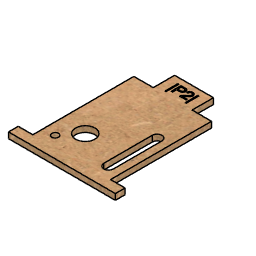
P2 (Autodesk Fusion 360 design; units mm, degrees)
Autodesk Fusion 360 part; units mm, degrees
note: some values were not read from the file. Set by a fixed rule: which sketch regions a step uses.
sketch "Esboço1" plane through (0, 0, 0) normal (0, 1, 0) x (1, 0, 0)
  line L0 (0, 0) -> (55, 0)
  line L1 (55, 0) -> (55, 5)
  line L2 (55, 5) -> (47.5, 5)
  line L3 (17.5, 68) -> (17.5, 57)
  line L4 (17.5, 57) -> (7.5, 57)
  line L5 (7.5, 57) -> (7.5, 5)
  line L6 (7.5, 5) -> (0, 5)
  line L7 (0, 5) -> (0, 0)
  circle A0 centre (13.5, 10.5) radius 1.75
  line L8 (43.5, 35.5) -> (43.5, 10.5)
  line L9 (38.5, 10.5) -> (38.5, 35.5)
  circle A1 centre (20.5, 19) radius 5
  line L10 (41, 68.4978) -> (41, 0)
  arc A2 (38.5, 10.5) -> (43.5, 10.5) centre (41, 10.5) ccw
  arc A3 (43.5, 35.5) -> (38.5, 35.5) centre (41, 35.5) ccw
  line L11 (37.5, 68) -> (37.5, 57)
  line L12 (37.5, 57) -> (47.5, 57)
  line L13 (17.5, 68) -> (37.5, 68)
  line L14 (47.5, 57) -> (47.5, 5)
  dimension "d1" = 55
  dimension "d2" = 5
  dimension "d4" = 10
  dimension "d8" = 3.5
  dimension "d10" = 6
  dimension "d18" = 10
  dimension "d38" = 5.5
  dimension "d39" = 7.5
  dimension "d41" = 11
  dimension "d42" = 52
  dimension "d45" = 20.5
  dimension "d46" = 2.5
  dimension "d47" = 5.5
  dimension "d48" = 5
  dimension "d49" = 25
  dimension "d50" = 2.5
  dimension "d51" = 8.5
  dimension "d54" = 11
  dimension "d55" = 10
  dimension "d56" = 20
  dimension "d57" = 52
  dimension "d58" = 4
  constraint coincident L0.start L7.end
  constraint horizontal L0
  constraint perpendicular L0 L1
  constraint perpendicular L1 L2
  constraint perpendicular L3 L4
  constraint perpendicular L4 L5
  constraint perpendicular L5 L6
  constraint perpendicular L0 L7
  constraint vertical L8
  constraint vertical L9
  constraint collinear L2 L6
  constraint vertical L10
  constraint coincident L0 L10.end
  constraint coincident L10 A2.centre
  constraint coincident L10 A3.centre
  constraint perpendicular L11 L13
  constraint perpendicular L2 L14
  measures "d1" distance of L0.start L0.end
  measures "d2" distance of L0.end L1.end
  measures "d4" distance of L3.end L4.end
  measures "d8" diameter of A0
  measures "d10" distance of L5 A0.centre
  measures "d18" diameter of A1
  measures "d38" distance of L6 A0.centre
  measures "d39" distance of L5.end L6.end
  measures "d41" distance of L3.start L3.end
  measures "d42" distance of L4.end L5.end
  measures "d45" distance of A1.centre L10
  measures "d46" radius of A2
  measures "d47" distance of L2 A2.centre
  measures "d48" distance of L8 L9
  measures "d49" distance of L8.end L8.start
  measures "d50" radius of A3
  measures "d51" vertical distance of A1.centre A2.centre
  measures "d54" distance of L11.start L11.end
  measures "d55" distance of L11.end L12.end
  measures "d56" distance of L3.start L11.start
  measures "d57" distance of L2 L12
  measures "d58" distance of L8 L14
extrude "Extrusão1" add sketch "Esboço1" along normal blind 3 contours L0 L3 L4 L5 L6 L7 L9 L10 A2 A3 L11 L12 L13 | L0 L1 L2 L8 L10 A2 A3 L12 L14
sketch "Esboço2" plane through (0, 3, 0) normal (0, 1, 0) x (-1, 0, 0)
  line L0 (-38.5, -10.5) -> (-38.5, -35.5)
  line L1 (-43.5, -35.5) -> (-43.5, -10.5)
  circle A0 centre (-20.5, -19) radius 5
  circle A1 centre (-13.5, -10.5) radius 1.75
  line L2 (0, -5) -> (0, 0)
  line L3 (0, 0) -> (-55, 0)
  line L4 (-55, 0) -> (-55, -5)
  line L5 (-55, -5) -> (-47.5, -5)
  line L6 (-17.5, -68) -> (-17.5, -57)
  line L7 (-17.5, -57) -> (-7.5, -57)
  line L8 (-7.5, -57) -> (-7.5, -5)
  line L9 (-7.5, -5) -> (0, -5)
  line L10 (-22.5, -58.5) -> (-32.5, -58.5) construction
  line L11 (-32.5, -58.5) -> (-32.5, -66.5) construction
  line L12 (-32.5, -66.5) -> (-22.5, -66.5) construction
  line L13 (-22.5, -66.5) -> (-22.5, -58.5) construction
  arc A2 (-38.5, -10.5) -> (-43.5, -10.5) centre (-41, -10.5) ccw
  arc A3 (-43.5, -35.5) -> (-38.5, -35.5) centre (-41, -35.5) ccw
  line L14 (-47.5, -5) -> (-47.5, -57)
  line L15 (-47.5, -57) -> (-37.5, -57)
  line L16 (-37.5, -57) -> (-37.5, -68)
  line L17 (-37.5, -68) -> (-17.5, -68)
  dimension "d25" = 5
  dimension "d59" = 5
  dimension "d60" = 5
  dimension "d61" = 1.5
  dimension "d62" = 1.5
  text T0 "|P2|" font "Arial" height 5 align centre middle in box 10 x 8 at (-22.5, -58.5) x (-1, 0) y (0, -1) spacing 1
  measures "d59" distance of L6 L13
  measures "d60" distance of L11 L16
  measures "d61" distance of L12 L17
  measures "d62" distance of L7 L10
extrude "Extrusão2" cut sketch "Esboço2" against normal blind 1 text T0
